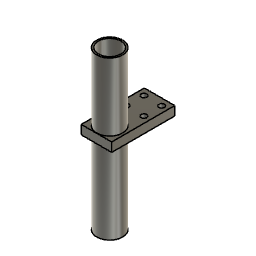
pH Sensor Guide Tube (Autodesk Fusion 360 design; units mm, degrees)
Autodesk Fusion 360 part; units mm, degrees
sketch "Sketch1" plane through (0, 0, 0) normal (0, 0, 1) x (1, 0, 0)
  circle A0 centre (0, 0) radius 10
  circle A1 centre (0, 0) radius 11.5
  dimension "d1" = 20
  dimension "d2" = 23
  constraint coincident A0.centre A1.centre
  constraint concentric A0 A1
  measures "d1" diameter of A0
  measures "d2" diameter of A1
extrude "Extrude1" add sketch "Sketch1" along normal blind 140
ref_plane "WorkPlane1" through (0, 0, 80) normal (0, 0, 1) x (1, 0, 0)
sketch "Sketch2" plane through (0, 0, 80) normal (0, 0, 1) x (1, 0, 0)
  line L0 (-11.5, 0) -> (11.5, 0)
  line L1 (11.5, 0) -> (11.5, 43)
  line L2 (11.5, 43) -> (-11.5, 43)
  line L3 (-11.5, 43) -> (-11.5, 0)
  circle A0 centre (0, 0) radius 11.5
  line L4 (0, 11.5) -> (-11.5, 11.5)
  circle A1 centre (-7.875, 24.5) radius 2.5
  circle A2 centre (-7.875, 40.25) radius 2.5
  line L5 (0, 11.5) -> (0, 43)
  circle A3 centre (7.875, 40.25) radius 2.5
  circle A4 centre (7.875, 24.5) radius 2.5
  line L6 (-13.5, 20.25) -> (13.5, 20.25)
  line L7 (13.5, 20.25) -> (13.5, 44.25)
  line L8 (13.5, 44.25) -> (-13.5, 44.25)
  line L9 (-13.5, 44.25) -> (-13.5, 20.25)
  point P0 (-11.5, 0)
  dimension "d6" = 23
  dimension "d7" = 3.625
  dimension "d8" = 13
  dimension "d9" = 5
  dimension "d10" = 5
  dimension "d11" = 15.75
  dimension "d12" = 2
  dimension "d13" = 24
  dimension "d14" = 2
  dimension "d15" = 4
  constraint horizontal L0
  constraint vertical L1
  constraint horizontal L2
  constraint vertical L3
  constraint coincident P0 L0.start
  constraint coincident A0.centre origin
  constraint coincident A0 L4.start
  constraint coincident L3 L4.end
  constraint tangent A0 L4
  constraint perpendicular L3 L4
  constraint midpoint L2 L5.end
  constraint symmetric A1 L5 A4
  constraint symmetric A2 L5 A3
  constraint horizontal L6
  constraint vertical L7
  constraint horizontal L8
  constraint vertical L9
  measures "d6" distance of L1 L3
  measures "d7" distance of L3 A1.centre
  measures "d8" distance of L4 A1.centre
  measures "d9" diameter of A1
  measures "d10" diameter of A2
  measures "d11" distance of A1.centre A2.centre
  measures "d12" distance of L3 L9
  measures "d13" distance of L6.end L7.end
  measures "d14" distance of L1 L7
  measures "d15" distance of A3.centre L8
extrude "Extrude2" add sketch "Sketch2" against normal blind 8 contours L3 A0 L4 | L1 A0 L5 L6 | L3 L4 L5 L6 | L1 L2 L5 L6 | L1 L2 L3 L6 L7 L8 L9 | L2 L3 L5 L6
sketch "Sketch3" plane through (0, 0, 80) normal (0, 0, 1) x (-1, 0, 0)
  circle A0 centre (7.875, -40.25) radius 2.5
  circle A1 centre (-7.875, -24.5) radius 2.5
  circle A2 centre (-7.875, -40.25) radius 2.5
  circle A3 centre (7.875, -24.5) radius 2.5
  line L0 (-11.5, 0) -> (-11.5, -20.25)
  line L1 (-11.5, -20.25) -> (-13.5, -20.25)
  line L2 (-13.5, -20.25) -> (-13.5, -44.25)
  line L3 (-13.5, -44.25) -> (13.5, -44.25)
  line L4 (13.5, -44.25) -> (13.5, -20.25)
  line L5 (13.5, -20.25) -> (11.5, -20.25)
  line L6 (11.5, -20.25) -> (11.5, 0)
  arc A4 (-11.5, 0) -> (11.5, 0) centre (0, 0) ccw
  line L7 (-13.5, -20.25) -> (13.5, -20.25)
  line L8 (13.5, -20.25) -> (13.5, 11.75)
  line L9 (13.5, 11.75) -> (-13.5, 11.75)
  line L10 (-13.5, 11.75) -> (-13.5, -20.25)
  circle A5 centre (0, 0) radius 11.5
  dimension "d18" = 32
  dimension "d19" = 27
  constraint horizontal L7
  constraint vertical L8
  constraint horizontal L9
  constraint vertical L10
  constraint coincident L1.end L2.start
  constraint concentric A4 A5
  measures "d18" distance of L4.end L8.end
  measures "d19" distance of L8 L10
extrude "Extrude3" add sketch "Sketch3" against normal blind 8 contours L0 L1 L5 L6 L7 L8 L9 L10 A5
move_face "MoveFace1" to x (1, 0, 0) y (0, 1, 0) z (0, 0, 1) at (0, -2, 0) 4 faces at (10.3626, 24.2511, 77.3333) (-5.3874, 24.2511, 77.3333) (-5.3874, 40.0011, 77.3333) (10.3626, 40.0011, 77.3333)
